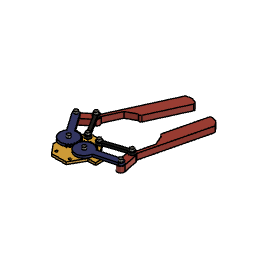
Edm exp 6.1 (Autodesk Fusion 360 design; units mm, degrees)
Autodesk Fusion 360 part; units mm, degrees
sketch "Sketch1" plane through (0, 0, 0) normal (0, 0, 1) x (1, 0, 0)
  line L0 (0, 0) -> (13.218, 0)
  line L1 (13.218, 0) -> (13.218, 17.4894)
  line L2 (0, 0) -> (-13.8101, -24.1272)
  line L3 (-13.8101, -24.1272) -> (-38.8101, -24.1272)
  line L4 (-38.8101, -24.1272) -> (-52.072, -8.3378)
  line L5 (-52.072, -8.3378) -> (-52.072, 21.6622)
  line L6 (-52.072, 21.6622) -> (-32.3728, 39.3428)
  line L7 (-32.3728, 39.3428) -> (-12.3728, 39.3428)
  line L8 (-12.3728, 39.3428) -> (2.5632, 17.4894)
  line L9 (2.5632, 17.4894) -> (13.218, 17.4894)
  dimension "d3" = 27.8
  dimension "d4" = 25
  dimension "d5" = 20.62
  dimension "d6" = 30
  dimension "d7" = 26.47
  dimension "d8" = 20
  dimension "d9" = 26.47
  constraint coincident L0.start L2.start
  constraint horizontal L0
  constraint perpendicular L0 L1
  constraint parallel L0 L3
  constraint perpendicular L3 L5
  constraint perpendicular L5 L7
  constraint parallel L0 L9
  measures "d3" distance of L0.start L2.end
  measures "d4" distance of L2.end L3.end
  measures "d5" distance of L3.end L4.end
  measures "d6" distance of L4.end L5.end
  measures "d7" distance of L5.end L6.end
  measures "d8" distance of L6.end L7.end
  measures "d9" distance of L7.end L8.end
extrude "Extrude1" add sketch "Sketch1" along normal blind 4 makes body 1
sketch "Sketch2" plane through (0, 0, 4) normal (0, 0, 1) x (-1, 0, 0)
  line L0 (0, 0) -> (-13.218, 0)
  line L1 (-13.218, 0) -> (-13.218, -17.4894)
  line L2 (-13.218, -17.4894) -> (-2.5632, -17.4894)
  line L3 (-2.5632, -17.4894) -> (12.3728, -39.3428)
  line L4 (12.3728, -39.3428) -> (32.3728, -39.3428)
  line L5 (32.3728, -39.3428) -> (52.072, -21.6622)
  line L6 (52.072, -21.6622) -> (52.072, 8.3378)
  line L7 (52.072, 8.3378) -> (38.8101, 24.1272)
  line L8 (38.8101, 24.1272) -> (13.8101, 24.1272)
  line L9 (13.8101, 24.1272) -> (0, 0)
  circle A0 centre (32.3728, -32.3428) radius 3
  circle A1 centre (12.3728, -32.3428) radius 3
  circle A2 centre (45.072, -11.6622) radius 3
  line L10 (15.982, -4.4894) -> (0.982, -4.4894)
  arc A3 (0.982, -4.4894) -> (0.982, -10.4894) centre (0.982, -7.4894) ccw
  line L11 (0.982, -10.4894) -> (15.982, -10.4894)
  arc A4 (15.982, -10.4894) -> (15.982, -4.4894) centre (15.982, -7.4894) ccw
  line L12 (15.982, -7.4894) -> (0.982, -7.4894) construction
  circle A5 centre (38.4114, 16.2325) radius 2
  circle A6 centre (15.0341, 16.2325) radius 2
  dimension "d14" = 6
  dimension "d18" = 6
  dimension "d21" = 6
  dimension "d24" = 4
  dimension "d25" = 4
  constraint tangent L10 A3
  constraint tangent A3 L11
  constraint parallel L10 L11
  constraint tangent L11 A4
  constraint tangent L10 A4
  constraint horizontal L12
  measures "d14" diameter of A0
  measures "d18" diameter of A1
  measures "d21" diameter of A2
  measures "d24" diameter of A5
  measures "d25" diameter of A6
extrude "Extrude2" cut sketch "Sketch2" against normal blind 100 contours A0 | A1 | A2 | L10 A3 L11 A4 | A5 | A6 bodies 1
sketch "Sketch1 (2)" plane through (0, 0, 4) normal (0, 0, 1) x (-1, 0, 0) in component "part 2"
  line L0 (0.982, -4.4894) -> (15.982, -4.4894)
  arc A0 (15.982, -10.4894) -> (15.982, -4.4894) centre (15.982, -7.4894) ccw
  line L1 (15.982, -10.4894) -> (0.982, -10.4894)
  arc A1 (0.982, -4.4894) -> (0.982, -10.4894) centre (0.982, -7.4894) ccw
  circle A2 centre (32.3728, -32.3428) radius 3
  circle A3 centre (38.4114, 16.2325) radius 2
  circle A4 centre (45.072, -11.6622) radius 3
  circle A5 centre (12.3728, -32.3428) radius 3
  circle A6 centre (15.0341, 16.2325) radius 2
  line L2 (0, 0) -> (-13.218, 0)
  line L3 (-13.218, 0) -> (-13.218, -17.4894)
  line L4 (-13.218, -17.4894) -> (-2.5632, -17.4894)
  line L5 (-2.5632, -17.4894) -> (12.3728, -39.3428)
  line L6 (12.3728, -39.3428) -> (32.3728, -39.3428)
  line L7 (32.3728, -39.3428) -> (52.072, -21.6622)
  line L8 (52.072, -21.6622) -> (52.072, 8.3378)
  line L9 (52.072, 8.3378) -> (38.8101, 24.1272)
  line L10 (38.8101, 24.1272) -> (13.8101, 24.1272)
  line L11 (13.8101, 24.1272) -> (0, 0)
  circle A7 centre (-20.8883, -20.403) radius 3
  circle A8 centre (-20.8883, 24.597) radius 3
  line L12 (-18.3881, 20.267) -> (-18.3881, -16.073)
  line L13 (-23.3885, 20.267) -> (-23.3885, -16.073)
  arc A9 (-23.3885, -16.073) -> (-18.3881, -16.073) centre (-20.8883, -20.403) ccw
  arc A10 (-18.3881, 20.267) -> (-23.3885, 20.267) centre (-20.8883, 24.597) ccw
  dimension "d28" = 10
  dimension "d29" = 6
  dimension "d30" = 45
  constraint concentric A7 A9
  constraint concentric A8 A10
  measures "d28" diameter of A9
  measures "d29" diameter of A7
  measures "d30" distance of A7.centre A8.centre
extrude "Extrude1'" add sketch "Sketch1 (2)" along normal blind 4 separate body contours L12 L13 A9 A10 makes body 2 in component "part 2"
sketch "Sketch1 (3)" plane through (0, 0, 0) normal (0, 0, 1) x (1, 0, 0) in component "part 3"
  circle A0 centre (35, 20) radius 3
  dimension "d34" = 6
  measures "d34" diameter of A0
extrude "Extrude1''" add sketch "Sketch1 (3)" along normal blind 18 separate body makes body 3 in component "part 3"
sketch "Sketch1 (4)" plane through (0, 0, 0) normal (0, 0, 1) x (1, 0, 0) in component "part 4"
  circle A0 centre (-75, 25.0348) radius 3
  circle A1 centre (-75, -26.97) radius 3
  line L0 (-79.9828, -26.556) -> (-79.9828, 10.8866)
  line L1 (-70.0172, -26.556) -> (-70.0175, 10.8865)
  arc A2 (-79.9828, -26.556) -> (-70.0172, -26.556) centre (-75, -26.97) ccw
  line L2 (-75.8493, 40.0067) -> (-75.8493, 41.5467)
  line L3 (-75.8493, 41.5467) -> (-75.5, 41.8612)
  line L4 (-75.5, 41.8612) -> (-75, 41.8612)
  line L5 (-74.1507, 40.0067) -> (-74.1507, 41.5467)
  line L6 (-74.1507, 41.5467) -> (-74.5, 41.8612)
  line L7 (-74.5, 41.8612) -> (-75, 41.8612)
  line L8 (-80.0939, 40.7643) -> (-79.838, 41.1585)
  line L9 (-79.838, 41.1585) -> (-79.355, 41.2879)
  line L10 (-78.872, 41.4173) -> (-79.355, 41.2879)
  line L11 (-79.6954, 39.2767) -> (-80.0939, 40.7643)
  line L12 (-78.4533, 41.2039) -> (-78.872, 41.4173)
  line L13 (-78.0547, 39.7164) -> (-78.4533, 41.2039)
  line L14 (-83.9914, 38.9099) -> (-83.8462, 39.3569)
  line L15 (-83.8462, 39.3569) -> (-83.4132, 39.6069)
  line L16 (-82.9802, 39.8569) -> (-83.4132, 39.6069)
  line L17 (-83.2214, 37.5762) -> (-83.9914, 38.9099)
  line L18 (-82.5205, 39.7592) -> (-82.9802, 39.8569)
  line L19 (-81.7505, 38.4255) -> (-82.5205, 39.7592)
  line L20 (-87.2762, 36.11) -> (-87.2516, 36.5793)
  line L21 (-87.2516, 36.5793) -> (-86.8981, 36.9329)
  line L22 (-86.5445, 37.2864) -> (-86.8981, 36.9329)
  line L23 (-86.1873, 35.021) -> (-87.2762, 36.11)
  line L24 (-86.0752, 37.311) -> (-86.5445, 37.2864)
  line L25 (-84.9862, 36.2221) -> (-86.0752, 37.311)
  line L26 (-89.7244, 32.5553) -> (-89.8221, 33.015)
  line L27 (-89.8221, 33.015) -> (-89.5721, 33.448)
  line L28 (-89.3221, 33.881) -> (-89.5721, 33.448)
  line L29 (-88.3907, 31.7853) -> (-89.7244, 32.5553)
  line L30 (-88.8751, 34.0262) -> (-89.3221, 33.881)
  line L31 (-87.5414, 33.2562) -> (-88.8751, 34.0262)
  line L32 (-91.1691, 28.4881) -> (-91.3825, 28.9068)
  line L33 (-91.3825, 28.9068) -> (-91.2531, 29.3898)
  line L34 (-91.1237, 29.8728) -> (-91.2531, 29.3898)
  line L35 (-89.6816, 28.0895) -> (-91.1691, 28.4881)
  line L36 (-90.7295, 30.1287) -> (-91.1237, 29.8728)
  line L37 (-89.242, 29.7301) -> (-90.7295, 30.1287)
  line L38 (-91.5119, 24.1855) -> (-91.8264, 24.5348)
  line L39 (-91.8264, 24.5348) -> (-91.8264, 25.0348)
  line L40 (-91.8264, 25.5348) -> (-91.8264, 25.0348)
  line L41 (-89.9719, 24.1855) -> (-91.5119, 24.1855)
  line L42 (-91.5119, 25.8841) -> (-91.8264, 25.5348)
  line L43 (-89.9719, 25.8841) -> (-91.5119, 25.8841)
  line L44 (-90.7295, 19.9409) -> (-91.1237, 20.1968)
  line L45 (-91.1237, 20.1968) -> (-91.2531, 20.6798)
  line L46 (-91.3825, 21.1628) -> (-91.2531, 20.6798)
  line L47 (-89.242, 20.3394) -> (-90.7295, 19.9409)
  line L48 (-91.1691, 21.5815) -> (-91.3825, 21.1628)
  line L49 (-89.6816, 21.9801) -> (-91.1691, 21.5815)
  line L50 (-88.8751, 16.0433) -> (-89.3221, 16.1886)
  line L51 (-89.3221, 16.1886) -> (-89.5721, 16.6216)
  line L52 (-89.8221, 17.0546) -> (-89.5721, 16.6216)
  line L53 (-87.5414, 16.8133) -> (-88.8751, 16.0433)
  line L54 (-89.7244, 17.5143) -> (-89.8221, 17.0546)
  line L55 (-88.3907, 18.2843) -> (-89.7244, 17.5143)
  line L56 (-86.0752, 12.7586) -> (-86.5445, 12.7832)
  line L57 (-86.5445, 12.7832) -> (-86.8981, 13.1367)
  line L58 (-87.2516, 13.4903) -> (-86.8981, 13.1367)
  line L59 (-84.9862, 13.8475) -> (-86.0752, 12.7586)
  line L60 (-87.2762, 13.9596) -> (-87.2516, 13.4903)
  line L61 (-86.1873, 15.0486) -> (-87.2762, 13.9596)
  line L62 (-82.5205, 10.3104) -> (-82.9802, 10.2127)
  line L63 (-82.9802, 10.2127) -> (-83.4132, 10.4627)
  line L64 (-83.8462, 10.7127) -> (-83.4132, 10.4627)
  line L65 (-81.7505, 11.6441) -> (-82.5205, 10.3104)
  line L66 (-83.9914, 11.1597) -> (-83.8462, 10.7127)
  line L67 (-83.2214, 12.4934) -> (-83.9914, 11.1597)
  arc A3 (-70.0175, 10.8865) -> (-74.1507, 40.0107) centre (-75, 25.0348) ccw
  arc A4 (-75.8493, 40.0107) -> (-78.0557, 39.7202) centre (-75, 25.0348) ccw
  arc A5 (-79.6964, 39.2806) -> (-81.7525, 38.429) centre (-75, 25.0348) ccw
  arc A6 (-83.2235, 37.5797) -> (-84.9891, 36.2249) centre (-75, 25.0348) ccw
  arc A7 (-86.1901, 35.0239) -> (-87.5449, 33.2583) centre (-75, 25.0348) ccw
  arc A8 (-88.3942, 31.7873) -> (-89.2458, 29.7312) centre (-75, 25.0348) ccw
  arc A9 (-89.6855, 28.0905) -> (-89.9759, 25.8841) centre (-75, 25.0348) ccw
  arc A10 (-89.9759, 24.1855) -> (-89.6855, 21.9791) centre (-75, 25.0348) ccw
  arc A11 (-89.2458, 20.3384) -> (-88.3942, 18.2823) centre (-75, 25.0348) ccw
  arc A12 (-87.5449, 16.8113) -> (-86.1901, 15.0457) centre (-75, 25.0348) ccw
  arc A13 (-84.9891, 13.8447) -> (-83.2235, 12.4899) centre (-75, 25.0348) ccw
  arc A14 (-81.7525, 11.6406) -> (-79.9828, 10.8866) centre (-75, 25.0348) ccw
  dimension "d37" = 30
  dimension "d38" = 6
  dimension "d39" = 10
  dimension "d40" = 6
  dimension "d47" = 150
  constraint concentric A0 A3
  constraint concentric A1 A2
  constraint vertical L0
  constraint vertical L2
  constraint coincident L5 A3.end
  constraint coincident L2 A4.start
  constraint concentric A3 A4
  constraint coincident L13 A4.end
  constraint coincident L11 A5.start
  constraint concentric A4 A5
  constraint coincident L19 A5.end
  constraint coincident L17 A6.start
  constraint concentric A5 A6
  constraint coincident L25 A6.end
  constraint coincident L23 A7.start
  constraint concentric A6 A7
  constraint coincident L31 A7.end
  constraint coincident L29 A8.start
  constraint concentric A7 A8
  constraint coincident L37 A8.end
  constraint coincident L35 A9.start
  constraint concentric A8 A9
  constraint coincident L43 A9.end
  constraint coincident L41 A10.start
  constraint concentric A9 A10
  constraint coincident L49 A10.end
  constraint coincident L47 A11.start
  constraint concentric A10 A11
  constraint coincident L55 A11.end
  constraint coincident L53 A12.start
  constraint concentric A11 A12
  constraint coincident L61 A12.end
  constraint coincident L59 A13.start
  constraint concentric A12 A13
  constraint coincident L67 A13.end
  constraint coincident L65 A14.start
  constraint concentric A13 A14
  measures "d37" diameter of A3
  measures "d38" diameter of A0
  measures "d39" diameter of A2
  measures "d40" diameter of A1
extrude "Extrude1'''" add sketch "Sketch1 (4)" along normal blind 4 separate body makes body 4 in component "part 4"
sketch "Sketch1 (5)" plane through (0, 0, 0) normal (0, 0, 1) x (1, 0, 0) in component "part5"
  line L0 (116.0946, -25) -> (116.0946, 0)
  arc A0 (116.0946, 0) -> (104.0946, 0) centre (110.0946, 0) ccw
  line L1 (104.0946, 0) -> (104.0946, -25)
  arc A1 (104.0946, -25) -> (116.0946, -25) centre (110.0946, -25) ccw
  line L2 (110.0946, -25) -> (110.0946, 0) construction
  line L3 (105.383, 3.715) -> (56.6674, 105.3923)
  line L4 (56.6674, 105.3923) -> (61.4274, 114.0729)
  line L5 (61.4274, 114.0729) -> (69.1698, 118.2421)
  line L6 (73.1717, 116.8329) -> (102.5535, 55.5083)
  arc A2 (73.1717, 116.8329) -> (69.1698, 118.2421) centre (70.4662, 115.5366) ccw
  line L7 (109.3973, 5.9593) -> (96.4347, 33.0143)
  line L8 (101.1442, 51.5065) -> (100.2424, 51.0744)
  line L9 (100.2424, 51.0744) -> (96.4347, 33.0143)
  arc A3 (101.1442, 51.5065) -> (102.5535, 55.5083) centre (99.848, 54.212) ccw
  dimension "d63" = 30
  dimension "d65" = 3
  constraint tangent L0 A0
  constraint tangent A0 L1
  constraint parallel L0 L1
  constraint tangent L1 A1
  constraint tangent L0 A1
  constraint vertical L2
  constraint coincident A0 L3.start
  constraint parallel L3 L6
  constraint coincident A0 L7.start
  constraint perpendicular L6 L8
  constraint tangent L6 A3
  constraint tangent L8 A3
  measures "d63" distance of L7.start L7.end
  measures "d65" radius of A3
extrude "Extrude1''''" add sketch "Sketch1 (5)" along normal blind 10 separate body makes body 5 in component "part5"
sketch "Sketch2 (2)" plane through (0, 0, 10) normal (0, 0, 1) x (-1, 0, 0) in component "part5"
  line L0 (-100.2424, -51.0744) -> (-101.1442, -51.5065)
  arc A0 (-101.1442, -51.5065) -> (-102.5535, -55.5083) centre (-99.848, -54.212) ccw
  line L1 (-102.5535, -55.5083) -> (-73.1717, -116.8329)
  arc A1 (-73.1717, -116.8329) -> (-69.1698, -118.2421) centre (-70.4662, -115.5366) ccw
  line L2 (-69.1698, -118.2421) -> (-61.4274, -114.0729)
  line L3 (-61.4274, -114.0729) -> (-56.6674, -105.3923)
  line L4 (-56.6674, -105.3923) -> (-105.383, -3.715)
  arc A2 (-105.383, -3.715) -> (-104.0946, 0) centre (-110.0946, 0) ccw
  line L5 (-104.0946, 0) -> (-104.0946, 25)
  arc A3 (-104.0946, 25) -> (-116.0946, 25) centre (-110.0946, 25) ccw
  line L6 (-116.0946, 25) -> (-116.0946, 0)
  arc A4 (-116.0946, 0) -> (-109.3973, -5.9593) centre (-110.0946, 0) ccw
  line L7 (-109.3973, -5.9593) -> (-96.4347, -33.0143)
  line L8 (-96.4347, -33.0143) -> (-100.2424, -51.0744)
  circle A5 centre (-110.0946, 0) radius 3
  circle A6 centre (-110.0946, 25) radius 3
  dimension "d70" = 6
  dimension "d71" = 6
  constraint concentric A2 A5
  constraint concentric A3 A6
  measures "d70" diameter of A5
  measures "d71" diameter of A6
extrude "Extrude2'" cut sketch "Sketch2 (2)" against normal blind 100 contours A5 | A6 bodies 5 in component "part5"
component "part 2" placed x (0.848048, 0.529919, 0) y (-0.529919, 0.848048, 0) z (0, 0, 1) at (-63.1215, 42.1331, 0)
component "part 3" placed x (0.819152, 0.573576, 0) y (-0.573576, 0.819152, 0) z (0, 0, 1) at (-92.0996, 17.8039, -6)
component "part 4" placed x (-0.819152, -0.573576, 0) y (0.573576, -0.819152, 0) z (0, 0, 1) at (-120.8678, -10.8487, 4)
component "part5" placed x (0.642788, -0.766044, 0) y (0.766044, 0.642788, 0) z (0, 0, 1) at (-126.5171, 154.6691, -6)
component "Component 6" placed x (1, 0, 0) y (0, 1, 0) z (0, 0, 1) at (0, 0, 0)
component "part 4" placed x (0.258819, -0.965926, 0) y (-0.965926, -0.258819, 0) z (0, 0, -1) at (29.6111, -58.4756, 8)
component "part 2" placed x (0.309017, -0.951057, 0) y (0.951057, 0.309017, 0) z (0, 0, 1) at (4.5654, 59.8096, 0)
component "part5" placed x (-0.978148, -0.207912, 0) y (-0.207912, 0.978148, 0) z (0, 0, -1) at (138.7417, 68.2928, 4)
component "part 3" placed x (0.848048, 0.529919, 0) y (-0.529919, 0.848048, 0) z (0, 0, 1) at (-75.3025, 34.9968, -6)
component "part 3" placed x (0.965926, 0.258819, 0) y (-0.258819, 0.965926, 0) z (0, 0, 1) at (7.6197, -7.428, -6)
component "part 3" placed x (0.951057, 0.309017, 0) y (-0.309017, 0.951057, 0) z (0, 0, 1) at (3.3181, 16.4119, -6)
component "part 3" placed x (0.819152, 0.573576, 0) y (-0.573576, 0.819152, 0) z (0, 0, 1) at (-62.2708, -24.796, -6)
component "part 3" placed x (0.965926, 0.258819, 0) y (-0.258819, 0.965926, 0) z (0, 0, 1) at (-42.6131, -20.8878, -6)
component "part 3" placed x (0.951057, 0.309017, 0) y (-0.309017, 0.951057, 0) z (0, 0, 1) at (-39.4795, 2.5061, -6)
component "part 3" placed x (0.848048, 0.529919, 0) y (-0.529919, 0.848048, 0) z (0, 0, 1) at (-51.4561, -3.1653, -6)
